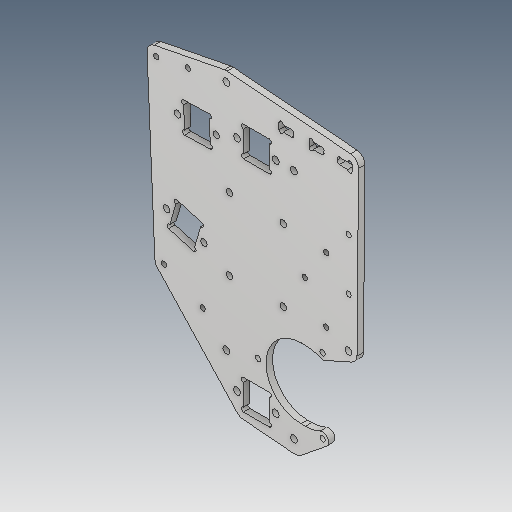
# Autodesk Inventor part: 2019スライダ側板02
Saved by Autodesk Inventor 2019.4 (Build 234330000, 330)
## iProperties
Created: 2018-05-19
Part Number: 2019スライダ側板02
Material: アルミニウム 2014-T4
Document SubType Name: Modeling
Designer: AzLIer
Density: 2.8 g/cm^3
Appearance: サテン
Mass: 80.0507 g
Surface Area: 220.985 cm^2
Volume: 28.5896 cm^3
Author: AzLIer
Autodesk Inventor part; units mm, degrees
(part 1 of 2)
ref_plane "YZ Plane" through (0, 0, 0) normal (1, 0, 0) x (0, 1, 0)
ref_plane "XZ Plane" through (0, 0, 0) normal (0, 1, 0) x (-1, 0, 0)
ref_plane "作業平面1" through (0, 0, 0) normal (0, 0, 1) x (1, 0, 0)
sketch "スケッチ1" plane through (0, 0, 0) normal (0, 0, 1) x (1, 0, 0)
  line L0 (0, 148) -> (2, 148) construction
  line L1 (2, 148) -> (2, 140) construction
  line L2 (2, 140) -> (0, 140) construction
  line L3 (0, 40) -> (0, 140) construction
  line L4 (0, 40) -> (2, 40) construction
  line L5 (2, 40) -> (2, 32) construction
  line L6 (2, 32) -> (0, 32) construction
  line L7 (0, 0) -> (0, 32) construction
  line L8 (25, 0) -> (0, 0) construction
  line L9 (25, 0) -> (25, 12) construction
  line L10 (25, 12) -> (23, 12) construction
  line L11 (23, 12) -> (23, 20) construction
  line L12 (23, 20) -> (25, 20) construction
  line L13 (25, 20) -> (25, 120) construction
  line L14 (25, 120) -> (23, 120) construction
  line L15 (23, 120) -> (23, 128) construction
  line L16 (23, 128) -> (25, 128) construction
  line L17 (25, 128) -> (25, 160) construction
  line L18 (0, 160) -> (25, 160) construction
  line L19 (0, 148) -> (0, 160) construction
  line L20 (-7.5, 150) -> (62.5, 150)
  line L21 (62.5, 150) -> (62.5, 10)
  line L22 (62.5, 10) -> (-7.5, 10)
  line L23 (-7.5, 10) -> (-7.5, 150)
  line L24 (5, -403.0972) -> (20, -403.0972) projected
  line L25 (5, -403.0972) -> (5, 396.9028) projected
  line L26 (20, 396.9028) -> (5, 396.9028) projected
  line L27 (20, -403.0972) -> (20, 396.9028) projected
  circle A0 centre (12.5, -388.0972) radius 1.5 projected
  circle A1 centre (12.5, -378.0972) radius 1.5 projected
  circle A2 centre (12.5, -398.0972) radius 1.5 projected
  circle A3 centre (12.5, 371.9028) radius 1.6 projected
  circle A4 centre (12.5, 391.9028) radius 1.6 projected
  circle A5 centre (12.5, 381.9028) radius 1.6 projected
  point P0 (2, 144)
  point P1 (23, 16)
  point P2 (-1.5, 144)
  point P3 (30, 16)
  point P4 (-1.5, 36)
  point P5 (30, 124)
  dimension "d0" = 70
  dimension "d1" = 140
  dimension "d2" = 6
  dimension "d3" = 6
  dimension "d4" = 3.5
  dimension "d5" = 6
  dimension "d7" = 20
  dimension "d8" = 20
  dimension "d167" = 10
  constraints: 8 end point, 2 horizontal alignment, 2 midpoint, 2 parallel, 2 vertical alignment, 1 horizontal, 1 perpendicular
  measures "d0" distance of L21.end L22.end
  measures "d1" distance of L20.end L21.end
  measures "d2" distance from line of L20 point (2, 144)
  measures "d3" distance from line of L22 point (23, 16)
  measures "d4" distance of point (-1.5, 144) point (2, 144)
  measures "d5" distance from line of point (-1.5, 144) L23
  measures "d7" vertical distance of point (2, 144) point (30, 124)
  measures "d8" vertical distance of point (-1.5, 36) point (30, 16)
  measures "d167" distance from line of L27 point (30, 16)
extrude "押し出し1" add sketch "スケッチ1" along normal blind 3 contours L20 L25 L22 L23 | L20 L27 L22 L25 | L20 L21 L22 L27
hole "穴1" at (-1.5, 144, 0) at (30, 16, 0) at (-1.5, 36, 0) at (30, 124, 0) direction (0, 0, 1) diameter 3.2 end through all
sketch "スケッチ2" plane through (0, 0, 3) normal (0, 0, 1) x (1, 0, 0)
  line L0 (23.3, 560) -> (23.3, -40) projected
  line L1 (-7.5, 10) -> (62.5, 10) projected
  point P0 (0, 0)
  point P1 (33.3, 40)
  dimension "d18" = 10
  dimension "d19" = 30
  measures "d18" distance from line of point (33.3, 40) L0
  measures "d19" distance from line of L1 point (33.3, 40)
hole "穴2" at (33.3, 40, 3) direction (0, 0, -1) diameter 20 end through all
sketch "スケッチ3" plane through (0, 0, 3) normal (0, 0, 1) x (1, 0, 0)
  circle A0 centre (33.3, 40) radius 10 projected
  circle A1 centre (-1.5, 36) radius 1.6 projected
  circle A2 centre (-1.5, 144) radius 1.6 projected
  circle A3 centre (30, 16) radius 1.6 projected
  circle A4 centre (30, 124) radius 1.6 projected
  line L0 (62.5, 150) -> (-7.5, 150) projected
  line L1 (-7.5, 150) -> (-7.5, 10) projected
  line L2 (-7.5, 10) -> (62.5, 10) projected
  line L3 (62.5, 10) -> (62.5, 150) projected
  line L4 (-7.5, 150) -> (-47.5, 150)
  line L5 (-47.5, 150) -> (-47.5, 10)
  line L6 (-47.5, 10) -> (-7.5, 10)
  line L7 (-7.5, 10) -> (-7.5, 150)
  point P0 (0, 0)
  dimension "d27" = 40
  constraints: 8 end point, 2 parallel, 1 horizontal, 1 perpendicular, 1 point on line
  measures "d27" distance of L6.end L5.end
extrude "押し出し2" add sketch "スケッチ3" against normal blind 3 contours L1 L6 L5 L4
sketch "スケッチ4" plane through (0, 0, 3) normal (0, 0, 1) x (1, 0, 0)
  circle A0 centre (33.3, 40) radius 10 projected
  circle A1 centre (-1.5, 36) radius 1.6 projected
  circle A2 centre (-1.5, 144) radius 1.6 projected
  circle A3 centre (30, 16) radius 1.6 projected
  circle A4 centre (30, 124) radius 1.6 projected
  line L0 (62.5, 150) -> (-47.5, 150) projected
  line L1 (-47.5, 150) -> (-47.5, 10) projected
  line L2 (-47.5, 10) -> (62.5, 10) projected
  line L3 (62.5, 10) -> (62.5, 150) projected
  line L4 (-11.5199, 142.1423) -> (-129.5092, 120.2671)
  line L5 (-131.6056, 104.3356) -> (-5.2401, 44.0714)
  circle A5 centre (-19.3858, 140.684) radius 1.6 projected
  circle A6 centre (-121.6432, 121.7254) radius 1.6 projected
  circle A7 centre (-106.8945, 124.4598) radius 1.6 projected
  circle A8 centre (-34.1345, 137.9496) radius 1.6 projected
  line L6 (-128.142, 112.8928) -> (-130.8764, 127.6414) projected
  line L7 (-128.142, 112.8928) -> (-10.1527, 134.768) projected
  line L8 (-12.8871, 149.5166) -> (-10.1527, 134.768) projected
  line L9 (-130.8764, 127.6414) -> (-12.8871, 149.5166) projected
  circle A9 centre (-12.461, 47.5151) radius 1.6 projected
  circle A10 centre (-124.3847, 100.8919) radius 1.6 projected
  circle A11 centre (-110.8456, 94.435) radius 1.6 projected
  circle A12 centre (-30.5132, 56.1243) radius 1.6 projected
  line L10 (-134.8341, 97.566) -> (-128.3772, 111.1051) projected
  line L11 (-134.8341, 97.566) -> (-8.4686, 37.3019) projected
  line L12 (-2.0117, 50.841) -> (-8.4686, 37.3019) projected
  line L13 (-128.3772, 111.1051) -> (-2.0117, 50.841) projected
  point P0 (0, 0)
  point P1 (-19.3858, 140.684)
  point P2 (-34.1345, 137.9496)
  point P3 (-30.5132, 56.1243)
  point P4 (-12.461, 47.5151)
  dimension "d147" = 15
  dimension "d148" = 20
  dimension "d150" = 8
  dimension "d151" = 8
  constraints: 4 end point, 4 midpoint, 4 point on line
  measures "d147" distance of point (-19.386, 140.684) point (-34.134, 137.95)
  measures "d148" distance of point (-12.461, 47.515) point (-30.513, 56.124)
  measures "d150" distance of point (-19.386, 140.684) L4.start
  measures "d151" distance of L5.end point (-12.461, 47.515)
hole "穴3" at (-34.1345, 137.9496, 3) at (-19.3858, 140.684, 3) at (-12.461, 47.5151, 3) at (-30.5132, 56.1243, 3) direction (0, 0, -1) diameter 2.459 end through all thread size "M3x0.5" class "6H" standard "ISO Metric profile"
sketch "スケッチ5" plane through (0, 0, 3) normal (0, 0, 1) x (1, 0, 0)
  arc A0 (43, 82) -> (43.866, 83.5) centre (43, 83) ccw projected
  line L0 (43, 82) -> (39, 82) projected
  arc A1 (37, 82) -> (39, 82) centre (38, 82) ccw projected
  line L1 (37, 82) -> (37, 85) projected
  arc A2 (39, 85) -> (37, 85) centre (38, 85) ccw projected
  line L2 (39, 85) -> (43, 85) projected
  arc A3 (43.866, 83.5) -> (43, 85) centre (43, 84) ccw projected
  arc A4 (57, 140) -> (55, 140) centre (56, 140) ccw projected
  line L3 (57, 140) -> (57, 137) projected
  arc A5 (55, 137) -> (57, 137) centre (56, 137) ccw projected
  line L4 (55, 137) -> (51, 137) projected
  arc A6 (50.134, 138.5) -> (51, 137) centre (51, 138) ccw projected
  arc A7 (51, 140) -> (50.134, 138.5) centre (51, 139) ccw projected
  line L5 (51, 140) -> (55, 140) projected
  arc A8 (25, 140) -> (23, 140) centre (24, 140) ccw projected
  line L6 (25, 140) -> (29, 140) projected
  arc A9 (29.866, 138.5) -> (29, 140) centre (29, 139) ccw projected
  arc A10 (29, 137) -> (29.866, 138.5) centre (29, 138) ccw projected
  line L7 (29, 137) -> (25, 137) projected
  arc A11 (23, 137) -> (25, 137) centre (24, 137) ccw projected
  line L8 (23, 137) -> (23, 140) projected
  arc A12 (39, 140) -> (37, 140) centre (38, 140) ccw projected
  line L9 (39, 140) -> (43, 140) projected
  arc A13 (43.866, 138.5) -> (43, 140) centre (43, 139) ccw projected
  arc A14 (43, 137) -> (43.866, 138.5) centre (43, 138) ccw projected
  line L10 (43, 137) -> (39, 137) projected
  arc A15 (37, 137) -> (39, 137) centre (38, 137) ccw projected
  line L11 (37, 137) -> (37, 140) projected
  arc A16 (57, 85) -> (55, 85) centre (56, 85) ccw projected
  line L12 (57, 85) -> (57, 82) projected
  arc A17 (55, 82) -> (57, 82) centre (56, 82) ccw projected
  line L13 (55, 82) -> (51, 82) projected
  arc A18 (50.134, 83.5) -> (51, 82) centre (51, 83) ccw projected
  arc A19 (51, 85) -> (50.134, 83.5) centre (51, 84) ccw projected
  line L14 (51, 85) -> (55, 85) projected
  arc A20 (29, 82) -> (29.866, 83.5) centre (29, 83) ccw projected
  line L15 (29, 82) -> (25, 82) projected
  arc A21 (23, 82) -> (25, 82) centre (24, 82) ccw projected
  line L16 (23, 82) -> (23, 85) projected
  arc A22 (25, 85) -> (23, 85) centre (24, 85) ccw projected
  line L17 (25, 85) -> (29, 85) projected
  arc A23 (29.866, 83.5) -> (29, 85) centre (29, 84) ccw projected
  circle A24 centre (-15, 140) radius 1.5 projected
  circle A25 centre (-15, 20) radius 1.5 projected
  line L18 (23.5, 121.4019) -> (23.5, 126.5981) projected
  arc A26 (25.4286, 126.9692) -> (23.5, 126.5981) centre (24.5, 126.5981) ccw projected
  arc A27 (25.4286, 121.0308) -> (25.4286, 126.9692) centre (25, 124) ccw projected
  arc A28 (23.5, 121.4019) -> (25.4286, 121.0308) centre (24.5, 121.4019) ccw projected
  line L19 (23.5, 13.4019) -> (23.5, 18.5981) projected
  arc A29 (25.4286, 18.9692) -> (23.5, 18.5981) centre (24.5, 18.5981) ccw projected
  arc A30 (25.4286, 13.0308) -> (25.4286, 18.9692) centre (25, 16) ccw projected
  arc A31 (23.5, 13.4019) -> (25.4286, 13.0308) centre (24.5, 13.4019) ccw projected
  circle A32 centre (-1.5, 144) radius 1.6 projected
  circle A33 centre (-1.5, 36) radius 1.6 projected
  line L20 (62.5, 150) -> (-22.5, 150) projected
  line L21 (-22.5, 150) -> (-22.5, 10) projected
  line L22 (-22.5, 10) -> (62.5, 10) projected
  line L23 (62.5, 10) -> (62.5, 150) projected
  point P0 (0, 0)
extrude "押し出し3" cut sketch "スケッチ5" against normal through all contours L3 A5 L4 A6 A7 L5 A4 | L6 A9 A10 L7 A11 L8 A8 | L9 A13 A14 L10 A15 L11 A12
sketch "スケッチ6" plane through (0, 0, 3) normal (0, 0, 1) x (1, 0, 0)
  circle A0 centre (33.3, 40) radius 10
  circle A1 centre (33.3, 40) radius 16
  circle A2 centre (55.3, 64) radius 1.6
  circle A3 centre (55.3, 16) radius 1.6
  line L0 (55.3, 64) -> (55.3, 16)
  circle A4 centre (55.3, 40) radius 1.6
  circle A5 centre (55.3, 40) radius 4.6
  point P0 (0, 0)
  dimension "d42" = 3.2
  dimension "d43" = 3.2
  dimension "d44" = 48
  dimension "d46" = 3.2
  dimension "d57" = 9.2
  dimension "d186" = 22
  constraints: 6 centre point, 2 end point, 1 coincident, 1 horizontal alignment, 1 midpoint, 1 vertical, 1 vertical alignment, 4 other
  measures "d42" diameter of A2
  measures "d43" diameter of A3
  measures "d44" distance of L0.end L0.start
  measures "d46" diameter of A4
  measures "d57" diameter of A5
  measures "d186" distance of A0.centre A4.centre
extrude "押し出し4" cut sketch "スケッチ6" against normal through all contours A2
sketch "スケッチ7" plane through (0, 0, 0) normal (0, 0, -1) x (-1, 0, 0)
  circle A0 centre (-25, 100.25) radius 1.25
  circle A1 centre (-25, 66.75) radius 1.25
  circle A2 centre (0, 100.25) radius 1.25
  circle A3 centre (0, 66.75) radius 1.5
  circle A4 centre (-25, 66.75) radius 1.5
  circle A5 centre (-25, 100.25) radius 1.5
  circle A6 centre (0, 100.25) radius 1.5
  circle A7 centre (0, 66.75) radius 1.5
  point P0 (0, 0)
  dimension "d52" = 3
  dimension "d53" = 3
  dimension "d54" = 3
  constraints: 8 centre point, 4 coincident, 1 concentric, 8 other
  measures "d52" diameter of A4
  measures "d53" diameter of A5
  measures "d54" diameter of A6
extrude "押し出し5" cut sketch "スケッチ7" against normal through all contours A0 | A1 | A2 | A3 | A4 | A5 | A6
sketch "スケッチ9" plane through (0, 0, 3) normal (0, 0, 1) x (1, 0, 0)
  circle A0 centre (55.4, 111) radius 1.25
  circle A1 centre (55.4, 87) radius 1.25
  point P0 (0, 0)
  dimension "d189" = 2.5
  dimension "d190" = 24
  constraints: 2 centre point, 1 equal radius, 1 vertical alignment, 1 other
  measures "d189" diameter of A1
  measures "d190" distance of A1.centre A0.centre
extrude "押し出し7" cut sketch "スケッチ9" against normal through all
sketch "スケッチ11" plane through (0, 0, 0) normal (0, 0, -1) x (-1, 0, 0)
  circle A0 centre (-33.3, 40) radius 10 projected
  circle A1 centre (-33.3, 53) radius 1.6
  circle A2 centre (-46.3, 40) radius 1.6
  circle A3 centre (-33.3, 27) radius 1.6
  circle A4 centre (-20.3, 40) radius 1.6
  line L0 (-46.3, 40) -> (-47.3, 40) construction
  line L1 (-46.3, 41.6) -> (-47.3, 41.6)
  line L2 (-47.3, 38.4) -> (-46.3, 38.4)
  arc A5 (-46.3, 38.4) -> (-46.3, 41.6) centre (-46.3, 40) ccw
  arc A6 (-47.3, 41.6) -> (-47.3, 38.4) centre (-47.3, 40) ccw
  line L3 (-33.3, 53) -> (-34.3, 53) construction
  line L4 (-33.3, 54.6) -> (-34.3, 54.6)
  line L5 (-34.3, 51.4) -> (-33.3, 51.4)
  arc A7 (-33.3, 51.4) -> (-33.3, 54.6) centre (-33.3, 53) ccw
  arc A8 (-34.3, 54.6) -> (-34.3, 51.4) centre (-34.3, 53) ccw
  line L6 (-20.3, 40) -> (-21.3, 40) construction
  line L7 (-20.3, 41.6) -> (-21.3, 41.6)
  line L8 (-21.3, 38.4) -> (-20.3, 38.4)
  arc A9 (-20.3, 38.4) -> (-20.3, 41.6) centre (-20.3, 40) ccw
  arc A10 (-21.3, 41.6) -> (-21.3, 38.4) centre (-21.3, 40) ccw
  line L9 (-33.3, 27) -> (-34.3, 27) construction
  line L10 (-33.3, 28.6) -> (-34.3, 28.6)
  line L11 (-34.3, 25.4) -> (-33.3, 25.4)
  arc A11 (-33.3, 25.4) -> (-33.3, 28.6) centre (-33.3, 27) ccw
  arc A12 (-34.3, 28.6) -> (-34.3, 25.4) centre (-34.3, 27) ccw
  line L12 (-33.3, 40) -> (-41.8797, 40) construction
  line L13 (-33.3, 44.2737) -> (-41.8797, 44.2737)
  line L14 (-41.8797, 35.7263) -> (-33.3, 35.7263)
  arc A13 (-33.3, 35.7263) -> (-33.3, 44.2737) centre (-33.3, 40) ccw
  arc A14 (-41.8797, 44.2737) -> (-41.8797, 35.7263) centre (-41.8797, 40) ccw
  point P0 (0, 0)
  point P1 (-46.8, 40)
  point P2 (-33.8, 53)
  point P3 (-20.8, 40)
  point P4 (-33.8, 27)
  point P5 (-37.5899, 40)
  dimension "d86" = 3.2
  dimension "d87" = 13
  dimension "d90" = 360
  dimension "d92" = 3.2
  dimension "d93" = 1
  constraints: 40 end point, 20 point on circle, 20 tangent, 14 centre point, 7 parallel, 5 midpoint, 3 equal length, 3 equal radius, 3 horizontal, 1 vertical alignment, 9 other
  measures "d86" diameter of A1
  measures "d87" distance of L3.start L12.start
  measures "d92" diameter of A6
  measures "d93" distance of L0.start L0.end
extrude "押し出し8" cut sketch "スケッチ11" against normal through all contours A14 A2 | A2 A14 | A2 L2 A6 L1 | A1 | A1 L5 A8 L4 | A3 | A3 L11 A12 L10 | A4 | A4 L8 A10 L7
sketch "スケッチ12" plane through (0, 0, 0) normal (0, 0, -1) x (-1, 0, 0)
  circle A0 centre (-33.3, 40) radius 10 projected
  line L0 (-28.9411, 31) -> (-38.6589, 31)
  line L1 (-28.9411, 49) -> (-38.6589, 49)
  arc A1 (-38.6589, 49) -> (-38.6589, 31) centre (-34.3, 40) ccw
  point P0 (0, 0)
  dimension "d96" = 18
  dimension "d98" = 1
  constraints: 4 end point, 4 point on circle, 2 horizontal, 1 centre point, 1 equal radius, 1 horizontal alignment, 1 parallel
  measures "d96" distance between parallel lines of L0 L1
  measures "d98" distance of A0.centre A1.centre
extrude "押し出し9" cut sketch "スケッチ12" against normal through all contours A0 L0 L1 | A0 L0 A1 L1
sketch "スケッチ13" plane through (0, 0, 0) normal (0, 0, -1) x (-1, 0, 0)
  line L0 (-28.9411, 31) -> (-37.6589, 31)
  arc A0 (-38.6589, 31) -> (-38.6589, 49) centre (-34.3, 40) ccw projected
  line L1 (-37.6589, 49) -> (-28.9411, 49)
  arc A1 (-37.6589, 31) -> (-28.9411, 31) centre (-33.3, 40) ccw
  arc A2 (-28.9411, 49) -> (-37.6589, 49) centre (-33.3, 40) ccw
  point P0 (0, 0)
  constraints: 4 end point, 4 point on circle, 3 centre point
extrude "押し出し10" add sketch "スケッチ13" against normal up to surface (3 mm away)
sketch "スケッチ14" plane through (0, 0, 0) normal (0, 0, -1) x (-1, 0, 0)
  arc A0 (-38.6589, 49) -> (-38.6589, 31) centre (-34.3, 40) ccw projected
  arc A1 (-28.9411, 31) -> (-28.9411, 49) centre (-33.3, 40) ccw projected
  line L0 (-33.3, 40) -> (-34.3, 40) construction
  line L1 (-33.3, 50) -> (-34.3, 50)
  line L2 (-34.3, 30) -> (-33.3, 30)
  arc A2 (-33.3, 30) -> (-33.3, 50) centre (-33.3, 40) ccw
  arc A3 (-34.3, 50) -> (-34.3, 30) centre (-34.3, 40) ccw
  line L3 (-33.3, 40) -> (-34.3, 40) construction
  line L4 (-33.3, 51.5) -> (-34.3, 51.5)
  line L5 (-34.3, 28.5) -> (-33.3, 28.5)
  arc A4 (-33.3, 28.5) -> (-33.3, 51.5) centre (-33.3, 40) ccw
  arc A5 (-34.3, 51.5) -> (-34.3, 28.5) centre (-34.3, 40) ccw
  circle A6 centre (-33.3, 40) radius 8 projected
  arc A7 (-44.2614, 39.1804) -> (-41.9476, 38.665) centre (-41.3284, 46.8961) ccw projected
  arc A8 (-41.9476, 38.665) -> (-41.8161, 37.9906) centre (-33.3, 40) ccw projected
  arc A9 (-41.8161, 37.9906) -> (-43.7672, 36.6441) centre (-38.1519, 30.5941) ccw projected
  arc A10 (-43.7672, 36.6441) -> (-43.4717, 35.8332) centre (-33.3, 40) ccw projected
  arc A11 (-43.4717, 35.8332) -> (-41.1118, 36.0581) centre (-43.0665, 44.0777) ccw projected
  arc A12 (-41.1118, 36.0581) -> (-40.7784, 35.4573) centre (-33.3, 40) ccw projected
  arc A13 (-40.7784, 35.4573) -> (-42.2179, 33.5738) centre (-35.0078, 29.5551) ccw projected
  arc A14 (-42.2179, 33.5738) -> (-41.6862, 32.8939) centre (-33.3, 40) ccw projected
  arc A15 (-41.6862, 32.8939) -> (-39.5113, 33.837) centre (-43.8486, 40.8601) ccw projected
  arc A16 (-39.5113, 33.837) -> (-39.0086, 33.3687) centre (-33.3, 40) ccw projected
  arc A17 (-39.0086, 33.3687) -> (-39.7956, 31.1326) centre (-31.6966, 29.5386) ccw projected
  arc A18 (-39.7956, 31.1326) -> (-39.0799, 30.6503) centre (-33.3, 40) ccw projected
  arc A19 (-39.0799, 30.6503) -> (-37.3028, 32.2193) centre (-43.5981, 37.5583) ccw projected
  arc A20 (-37.3028, 32.2193) -> (-36.68, 31.9292) centre (-33.3, 40) ccw projected
  arc A21 (-36.68, 31.9292) -> (-36.7375, 29.5593) centre (-28.5423, 30.5461) ccw projected
  arc A22 (-36.7375, 29.5593) -> (-35.9078, 29.3218) centre (-33.3, 40) ccw projected
  arc A23 (-35.9078, 29.3218) -> (-34.7025, 31.3631) centre (-42.3395, 34.4956) ccw projected
  arc A24 (-34.7025, 31.3631) -> (-34.0206, 31.2797) centre (-33.3, 40) ccw projected
  arc A25 (-34.0206, 31.2797) -> (-33.3429, 29.0081) centre (-25.8537, 32.479) ccw projected
  arc A26 (-33.3429, 29.0081) -> (-32.4804, 29.0386) centre (-33.3, 40) ccw projected
  arc A27 (-32.4804, 29.0386) -> (-31.965, 31.3524) centre (-40.1961, 31.9716) ccw projected
  arc A28 (-31.965, 31.3524) -> (-31.2906, 31.4839) centre (-33.3, 40) ccw projected
  arc A29 (-31.2906, 31.4839) -> (-29.9441, 29.5328) centre (-23.8941, 35.1481) ccw projected
  arc A30 (-29.9441, 29.5328) -> (-29.1332, 29.8283) centre (-33.3, 40) ccw projected
  arc A31 (-29.1332, 29.8283) -> (-29.3581, 32.1882) centre (-37.3777, 30.2335) ccw projected
  arc A32 (-29.3581, 32.1882) -> (-28.7573, 32.5216) centre (-33.3, 40) ccw projected
  arc A33 (-28.7573, 32.5216) -> (-26.8738, 31.0821) centre (-22.8551, 38.2922) ccw projected
  arc A34 (-26.8738, 31.0821) -> (-26.1939, 31.6138) centre (-33.3, 40) ccw projected
  arc A35 (-26.1939, 31.6138) -> (-27.137, 33.7887) centre (-34.1601, 29.4514) ccw projected
  arc A36 (-27.137, 33.7887) -> (-26.6687, 34.2914) centre (-33.3, 40) ccw projected
  arc A37 (-26.6687, 34.2914) -> (-24.4326, 33.5044) centre (-22.8386, 41.6034) ccw projected
  arc A38 (-24.4326, 33.5044) -> (-23.9503, 34.2201) centre (-33.3, 40) ccw projected
  arc A39 (-23.9503, 34.2201) -> (-25.5193, 35.9972) centre (-30.8583, 29.7019) ccw projected
  arc A40 (-25.5193, 35.9972) -> (-25.2292, 36.62) centre (-33.3, 40) ccw projected
  arc A41 (-25.2292, 36.62) -> (-22.8593, 36.5625) centre (-23.8461, 44.7577) ccw projected
  arc A42 (-22.8593, 36.5625) -> (-22.6218, 37.3922) centre (-33.3, 40) ccw projected
  arc A43 (-22.6218, 37.3922) -> (-24.6631, 38.5975) centre (-27.7956, 30.9605) ccw projected
  arc A44 (-24.6631, 38.5975) -> (-24.5797, 39.2794) centre (-33.3, 40) ccw projected
  arc A45 (-24.5797, 39.2794) -> (-22.3081, 39.9571) centre (-25.779, 47.4463) ccw projected
  arc A46 (-22.3081, 39.9571) -> (-22.3386, 40.8196) centre (-33.3, 40) ccw projected
  arc A47 (-22.3386, 40.8196) -> (-24.6524, 41.335) centre (-25.2716, 33.1039) ccw projected
  arc A48 (-24.6524, 41.335) -> (-24.7839, 42.0094) centre (-33.3, 40) ccw projected
  arc A49 (-24.7839, 42.0094) -> (-22.8328, 43.3559) centre (-28.4481, 49.4059) ccw projected
  arc A50 (-22.8328, 43.3559) -> (-23.1283, 44.1668) centre (-33.3, 40) ccw projected
  arc A51 (-23.1283, 44.1668) -> (-25.4882, 43.9419) centre (-23.5335, 35.9223) ccw projected
  arc A52 (-25.4882, 43.9419) -> (-25.8216, 44.5427) centre (-33.3, 40) ccw projected
  arc A53 (-25.8216, 44.5427) -> (-24.3821, 46.4262) centre (-31.5922, 50.4449) ccw projected
  arc A54 (-24.3821, 46.4262) -> (-24.9138, 47.1061) centre (-33.3, 40) ccw projected
  arc A55 (-24.9138, 47.1061) -> (-27.0887, 46.163) centre (-22.7514, 39.1399) ccw projected
  arc A56 (-27.0887, 46.163) -> (-27.5914, 46.6313) centre (-33.3, 40) ccw projected
  arc A57 (-27.5914, 46.6313) -> (-26.8044, 48.8674) centre (-34.9034, 50.4614) ccw projected
  arc A58 (-26.8044, 48.8674) -> (-27.5201, 49.3497) centre (-33.3, 40) ccw projected
  arc A59 (-27.5201, 49.3497) -> (-29.2972, 47.7807) centre (-23.0019, 42.4417) ccw projected
  arc A60 (-29.2972, 47.7807) -> (-29.92, 48.0708) centre (-33.3, 40) ccw projected
  arc A61 (-29.92, 48.0708) -> (-29.8625, 50.4407) centre (-38.0577, 49.4539) ccw projected
  arc A62 (-29.8625, 50.4407) -> (-30.6922, 50.6782) centre (-33.3, 40) ccw projected
  arc A63 (-30.6922, 50.6782) -> (-31.8975, 48.6369) centre (-24.2605, 45.5044) ccw projected
  arc A64 (-31.8975, 48.6369) -> (-32.5794, 48.7203) centre (-33.3, 40) ccw projected
  arc A65 (-32.5794, 48.7203) -> (-33.2571, 50.9919) centre (-40.7463, 47.521) ccw projected
  arc A66 (-33.2571, 50.9919) -> (-34.1196, 50.9614) centre (-33.3, 40) ccw projected
  arc A67 (-34.1196, 50.9614) -> (-34.635, 48.6476) centre (-26.4039, 48.0284) ccw projected
  arc A68 (-34.635, 48.6476) -> (-35.3094, 48.5161) centre (-33.3, 40) ccw projected
  arc A69 (-35.3094, 48.5161) -> (-36.6559, 50.4672) centre (-42.7059, 44.8519) ccw projected
  arc A70 (-36.6559, 50.4672) -> (-37.4668, 50.1717) centre (-33.3, 40) ccw projected
  arc A71 (-37.4668, 50.1717) -> (-37.2419, 47.8118) centre (-29.2223, 49.7665) ccw projected
  arc A72 (-37.2419, 47.8118) -> (-37.8427, 47.4784) centre (-33.3, 40) ccw projected
  arc A73 (-37.8427, 47.4784) -> (-39.7262, 48.9179) centre (-43.7449, 41.7078) ccw projected
  arc A74 (-39.7262, 48.9179) -> (-40.4061, 48.3862) centre (-33.3, 40) ccw projected
  arc A75 (-40.4061, 48.3862) -> (-39.463, 46.2113) centre (-32.4399, 50.5486) ccw projected
  arc A76 (-39.463, 46.2113) -> (-39.9313, 45.7086) centre (-33.3, 40) ccw projected
  arc A77 (-39.9313, 45.7086) -> (-42.1674, 46.4956) centre (-43.7614, 38.3966) ccw projected
  arc A78 (-42.1674, 46.4956) -> (-42.6497, 45.7799) centre (-33.3, 40) ccw projected
  arc A79 (-42.6497, 45.7799) -> (-41.0807, 44.0028) centre (-35.7417, 50.2981) ccw projected
  arc A80 (-41.0807, 44.0028) -> (-41.3708, 43.38) centre (-33.3, 40) ccw projected
  arc A81 (-41.3708, 43.38) -> (-43.7407, 43.4375) centre (-42.7539, 35.2423) ccw projected
  arc A82 (-43.7407, 43.4375) -> (-43.9782, 42.6078) centre (-33.3, 40) ccw projected
  arc A83 (-43.9782, 42.6078) -> (-41.9369, 41.4025) centre (-38.8044, 49.0395) ccw projected
  arc A84 (-41.9369, 41.4025) -> (-42.0203, 40.7206) centre (-33.3, 40) ccw projected
  arc A85 (-42.0203, 40.7206) -> (-44.2919, 40.0429) centre (-40.821, 32.5537) ccw projected
  arc A86 (-44.2919, 40.0429) -> (-44.2614, 39.1804) centre (-33.3, 40) ccw projected
  point P0 (0, 0)
  point P1 (-33.8, 40)
  point P2 (-33.8, 40)
  dimension "d191" = 23
  dimension "d192" = 1
  constraints: 16 end point, 8 point on circle, 8 tangent, 4 centre point, 2 horizontal, 2 midpoint, 2 parallel, 1 concentric
  measures "d191" diameter of A5
  measures "d192" distance of L0.start L3.end
extrude "押し出し12" cut sketch "スケッチ14" against normal through all contours A3 A71 A72 A73 A0 | A73 A72 A71 A3 A69 A68 A67 L1 A2 A65 A64 A63 A61 A60 A59 A1 A57 A56 A55 A53 A52 A51 A49 A48 A47 A45 A44 A43 A41 A40 A39 A37 A36 A35 A33 A32 A31 A29 A28 A27 L2 A25 A24 A23 A21 A20 A19 A0 A17 A16 A15 A13 A12 A11 A9 A8 A7 A86 A85 A84 A83 A81 A80 A79 A77 A76 A75 | A75 A76 A77 A0 | A3 A67 A68 A69 | A79 A80 A81 A0 | A83 A84 A85 A86 A7 A8 A9 A0 | A2 A63 A64 A65 | A11 A12 A13 A0 | A2 A1 A59 A60 A61 | A15 A16 A17 A0 | A1 A55 A56 A57 | A19 A20 A21 A3 | A1 A51 A52 A53 | A23 A24 A25 L2 A3 | A1 A47 A48 A49 | A1 A43 A44 A45 | A27 A28 A29 A2 | A1 A39 A40 A41 | A31 A32 A33 A1 A2 | A1 A35 A36 A37 | A6
sketch "スケッチ15" plane through (0, 0, 0) normal (0, 0, -1) x (-1, 0, 0)
  line L0 (47.5, 150) -> (-62.5, 150) projected
  line L1 (-62.5, 150) -> (-62.5, 10) projected
  line L2 (-62.5, 10) -> (47.5, 10) projected
  line L3 (47.5, 10) -> (47.5, 150) projected
  line L4 (14.8879, 112.0622) -> (15.4057, 128.0538) construction
  arc A0 (14.7909, 109.0638) -> (17.8864, 111.9651) centre (14.8879, 112.0622) ccw
  arc A1 (18.4041, 127.9567) -> (15.5028, 131.0523) centre (15.4057, 128.0538) ccw
  arc A2 (19.384, 150) -> (47.5, 25.9287) centre (155.0735, 115.5275) ccw construction
  line L5 (17.9187, 112.9646) -> (20.9172, 112.8675)
  line L6 (20.9819, 114.8665) -> (21.3055, 124.8612)
  line L7 (21.3702, 126.8602) -> (18.3718, 126.9573)
  arc A3 (20.9172, 112.8675) -> (20.9819, 114.8665) centre (20.9495, 113.867) ccw
  arc A4 (21.3055, 124.8612) -> (21.3702, 126.8602) centre (21.3378, 125.8607) ccw
  line L8 (17.8864, 111.9651) -> (17.9187, 112.9646)
  line L9 (18.3718, 126.9573) -> (18.4041, 127.9567)
  line L10 (21.1437, 119.8638) -> (15.1468, 120.058) construction
  line L11 (14.7909, 109.0638) -> (15.5028, 131.0523)
  circle A5 centre (24.1421, 119.7668) radius 1.5
  arc A6 (11.8895, 112.1593) -> (14.7909, 109.0638) centre (14.8879, 112.0622) ccw
  arc A7 (15.5028, 131.0523) -> (12.4073, 128.1509) centre (15.4057, 128.0538) ccw
  line L12 (11.9219, 113.1588) -> (8.9234, 113.2558)
  line L13 (8.9882, 115.2548) -> (9.3118, 125.2496)
  line L14 (9.3765, 127.2485) -> (12.3749, 127.1514)
  arc A8 (8.9882, 115.2548) -> (8.9234, 113.2558) centre (8.9558, 114.2553) ccw
  arc A9 (9.3765, 127.2485) -> (9.3118, 125.2496) centre (9.3441, 126.249) ccw
  line L15 (11.8895, 112.1593) -> (11.9219, 113.1588)
  line L16 (12.3749, 127.1514) -> (12.4073, 128.1509)
  line L17 (9.15, 120.2522) -> (15.1468, 120.058) construction
  circle A10 centre (6.1515, 120.3493) radius 1.5
  line L18 (24.4121, 84.9889) -> (21.5304, 84.1547)
  line L19 (26.3587, 78.265) -> (20.5953, 76.5966) construction
  line L20 (27.749, 73.4622) -> (24.9683, 83.0678)
  line L21 (14.832, 74.9281) -> (20.5953, 76.5966) construction
  arc A11 (28.3052, 71.5411) -> (27.749, 73.4622) centre (28.0271, 72.5017) ccw
  line L22 (25.4235, 70.7069) -> (28.3052, 71.5411)
  arc A12 (23.6542, 66.0304) -> (25.7016, 69.7463) centre (22.8199, 68.9121) ccw
  arc A13 (24.9683, 83.0678) -> (24.4121, 84.9889) centre (24.6902, 84.0284) ccw
  line L23 (15.7671, 82.4862) -> (15.489, 83.4468)
  arc A14 (17.5364, 87.1627) -> (15.489, 83.4468) centre (18.3707, 84.281) ccw
  arc A15 (21.2524, 85.1153) -> (17.5364, 87.1627) centre (18.3707, 84.281) ccw
  line L24 (19.6602, 69.0384) -> (16.7785, 68.2042)
  line L25 (25.7016, 69.7463) -> (25.4235, 70.7069)
  arc A16 (19.9383, 68.0779) -> (23.6542, 66.0304) centre (22.8199, 68.9121) ccw
  line L26 (22.8199, 68.9121) -> (18.3707, 84.281) construction
  line L27 (23.6542, 66.0304) -> (17.5364, 87.1627)
  line L28 (19.9383, 68.0779) -> (19.6602, 69.0384)
  circle A17 centre (29.2403, 79.0993) radius 1.5
  line L29 (21.5304, 84.1547) -> (21.2524, 85.1153)
  line L30 (12.8854, 81.652) -> (15.7671, 82.4862)
  line L31 (16.2223, 70.1253) -> (13.4416, 79.7309)
  arc A18 (12.8854, 81.652) -> (13.4416, 79.7309) centre (13.1635, 80.6914) ccw
  circle A19 centre (11.9503, 74.0939) radius 1.5
  arc A20 (16.2223, 70.1253) -> (16.7785, 68.2042) centre (16.5004, 69.1647) ccw
  line L32 (17.9187, 112.9646) -> (11.9219, 113.1588)
  line L33 (18.3718, 126.9573) -> (12.3749, 127.1514)
  line L34 (21.5304, 84.1547) -> (15.7671, 82.4862)
  line L35 (25.4235, 70.7069) -> (19.6602, 69.0384)
  arc A21 (201.0636, 258.3032) -> (63.0248, -2.9083) centre (155.0735, 115.5275) ccw projected
  line L36 (128.3772, 111.1051) -> (2.0117, 50.841) projected
  point P0 (0, 0)
  dimension "d130" = 140
  dimension "d131" = 16
  dimension "d132" = 3
  dimension "d133" = 1
  dimension "d134" = 3
  dimension "d135" = 14
  dimension "d137" = 3
  dimension "d138" = 3
  dimension "d141" = 18
  dimension "d152" = 54
  constraints: 68 end point, 35 point on circle, 22 point on line, 21 centre point, 12 symmetric about line, 5 tangent, 4 midpoint, 4 parallel, 4 perpendicular, 2 collinear, 1 concentric, 1 equal radius, 59 other
  measures "d130" radius of A2
  measures "d131" distance of L4.start L4.end
  measures "d132" radius of A0
  measures "d133" radius of A3
  measures "d134" distance of L5.start L5.end
  measures "d135" distance between parallel lines of L7 L5
  measures "d137" diameter of A5
  measures "d138" distance of L10.start A5.centre
extrude "押し出し13" cut sketch "スケッチ15" against normal through all contours A21 A10 | A10 A21 | A21 A19 | A19 A21 | L32 L12 A8 L13 A9 L14 L33 L11 | L11 L33 L7 A4 L6 A3 L5 L32 | A5 | A13 L20 A11 L22 L35 L27 L34 L18 | L27 L35 L24 A20 L31 A18 L30 L34 | A17
sketch "スケッチ18" plane through (0, 0, 3) normal (0, 0, 1) x (1, 0, 0)
  line L0 (-24.4121, 84.9889) -> (-12.8854, 81.652) projected
  arc A0 (-13.4416, 79.7309) -> (-12.8854, 81.652) centre (-13.1635, 80.6914) ccw projected
  line L1 (-13.4416, 79.7309) -> (-16.2223, 70.1253) projected
  arc A1 (-16.7785, 68.2042) -> (-16.2223, 70.1253) centre (-16.5004, 69.1647) ccw projected
  line L2 (-16.7785, 68.2042) -> (-28.3052, 71.5411) projected
  arc A2 (-27.749, 73.4622) -> (-28.3052, 71.5411) centre (-28.0271, 72.5017) ccw projected
  line L3 (-27.749, 73.4622) -> (-24.9683, 83.0678) projected
  arc A3 (-24.4121, 84.9889) -> (-24.9683, 83.0678) centre (-24.6902, 84.0284) ccw projected
  circle A4 centre (-11.9503, 74.0939) radius 1.5 projected
  circle A5 centre (-6.1515, 120.3493) radius 1.5 projected
  circle A6 centre (-24.1421, 119.7668) radius 1.5 projected
  circle A7 centre (-29.2403, 79.0993) radius 1.5 projected
  arc A8 (-9.3118, 125.2496) -> (-9.3765, 127.2485) centre (-9.3441, 126.249) ccw projected
  line L4 (-9.3118, 125.2496) -> (-8.9882, 115.2548) projected
  arc A9 (-8.9234, 113.2558) -> (-8.9882, 115.2548) centre (-8.9558, 114.2553) ccw projected
  line L5 (-8.9234, 113.2558) -> (-20.9172, 112.8675) projected
  arc A10 (-20.9819, 114.8665) -> (-20.9172, 112.8675) centre (-20.9495, 113.867) ccw projected
  line L6 (-20.9819, 114.8665) -> (-21.3055, 124.8612) projected
  arc A11 (-21.3702, 126.8602) -> (-21.3055, 124.8612) centre (-21.3378, 125.8607) ccw projected
  line L7 (-21.3702, 126.8602) -> (-9.3765, 127.2485) projected
  arc A12 (34.3, 25.4) -> (34.3, 28.6) centre (34.3, 27) ccw projected
  line L8 (34.3, 25.4) -> (33.3, 25.4) projected
  arc A13 (33.3, 28.6) -> (33.3, 25.4) centre (33.3, 27) ccw projected
  line L9 (33.3, 28.6) -> (34.3, 28.6) projected
  arc A14 (34.3, 51.4) -> (34.3, 54.6) centre (34.3, 53) ccw projected
  line L10 (34.3, 51.4) -> (33.3, 51.4) projected
  arc A15 (33.3, 54.6) -> (33.3, 51.4) centre (33.3, 53) ccw projected
  line L11 (33.3, 54.6) -> (34.3, 54.6) projected
  arc A16 (21.3, 38.4) -> (21.3, 41.6) centre (21.3, 40) ccw projected
  line L12 (21.3, 38.4) -> (20.3, 38.4) projected
  arc A17 (20.3, 41.6) -> (20.3, 38.4) centre (20.3, 40) ccw projected
  line L13 (20.3, 41.6) -> (21.3, 41.6) projected
  arc A18 (47.3, 38.4) -> (47.3, 41.6) centre (47.3, 40) ccw projected
  line L14 (47.3, 38.4) -> (46.3, 38.4) projected
  arc A19 (46.3, 41.6) -> (46.3, 38.4) centre (46.3, 40) ccw projected
  line L15 (46.3, 41.6) -> (47.3, 41.6) projected
  circle A20 centre (55.4, 111) radius 1.25 projected
  circle A21 centre (25, 100.25) radius 1.5 projected
  circle A22 centre (0, 66.75) radius 1.5 projected
  circle A23 centre (25, 66.75) radius 1.5 projected
  circle A24 centre (0, 100.25) radius 1.5 projected
  circle A25 centre (55.3, 64) radius 1.6 projected
  line L16 (23, 137) -> (23, 140) projected
  arc A26 (25, 140) -> (23, 140) centre (24, 140) ccw projected
  line L17 (25, 140) -> (29, 140) projected
  arc A27 (29.866, 138.5) -> (29, 140) centre (29, 139) ccw projected
  arc A28 (29, 137) -> (29.866, 138.5) centre (29, 138) ccw projected
  line L18 (29, 137) -> (25, 137) projected
  arc A29 (23, 137) -> (25, 137) centre (24, 137) ccw projected
  line L19 (51, 140) -> (55, 140) projected
  arc A30 (57, 140) -> (55, 140) centre (56, 140) ccw projected
  line L20 (57, 140) -> (57, 137) projected
  arc A31 (55, 137) -> (57, 137) centre (56, 137) ccw projected
  line L21 (55, 137) -> (51, 137) projected
  arc A32 (50.134, 138.5) -> (51, 137) centre (51, 138) ccw projected
  arc A33 (51, 140) -> (50.134, 138.5) centre (51, 139) ccw projected
  line L22 (37, 137) -> (37, 140) projected
  arc A34 (39, 140) -> (37, 140) centre (38, 140) ccw projected
  line L23 (39, 140) -> (43, 140) projected
  arc A35 (43.866, 138.5) -> (43, 140) centre (43, 139) ccw projected
  arc A36 (43, 137) -> (43.866, 138.5) centre (43, 138) ccw projected
  line L24 (43, 137) -> (39, 137) projected
  arc A37 (37, 137) -> (39, 137) centre (38, 137) ccw projected
  circle A38 centre (-12.461, 47.5151) radius 1.2295 projected
  circle A39 centre (-34.1345, 137.9496) radius 1.2295 projected
  circle A40 centre (-19.3858, 140.684) radius 1.2295 projected
  circle A41 centre (-30.5132, 56.1243) radius 1.2295 projected
  circle A42 centre (-1.5, 36) radius 1.6 projected
  circle A43 centre (-1.5, 144) radius 1.6 projected
  circle A44 centre (30, 16) radius 1.6 projected
  circle A45 centre (30, 124) radius 1.6 projected
  line L25 (62.5, 150) -> (-47.5, 150) projected
  line L26 (-47.5, 150) -> (-47.5, 10) projected
  line L27 (-47.5, 10) -> (62.5, 10) projected
  line L28 (62.5, 10) -> (62.5, 150) projected
  arc A46 (34.3, 30) -> (34.3, 50) centre (34.3, 40) ccw projected
  arc A47 (33.3, 50) -> (33.3, 30) centre (33.3, 40) ccw projected
  line L29 (20, -348.9108) -> (5, -348.9108) projected
  line L30 (20, -348.9108) -> (20, 451.0892) projected
  line L31 (5, 451.0892) -> (20, 451.0892) projected
  line L32 (5, -348.9108) -> (5, 451.0892) projected
  circle A48 centre (12.5, -333.9108) radius 1.5 projected
  circle A49 centre (12.5, -323.9108) radius 1.5 projected
  circle A50 centre (12.5, -343.9108) radius 1.5 projected
  circle A51 centre (12.5, 426.0892) radius 1.6 projected
  circle A52 centre (12.5, 446.0892) radius 1.6 projected
  circle A53 centre (12.5, 436.0892) radius 1.6 projected
  line L33 (6.5, 131) -> (18.5, 131)
  line L34 (18.5, 129) -> (18.5, 119)
  line L35 (18.5, 117) -> (6.5, 117)
  line L36 (6.5, 119) -> (6.5, 129)
  arc A54 (6.5, 131) -> (6.5, 129) centre (6.5, 130) ccw
  arc A55 (6.5, 119) -> (6.5, 117) centre (6.5, 118) ccw
  arc A56 (18.5, 129) -> (18.5, 131) centre (18.5, 130) ccw
  arc A57 (18.5, 117) -> (18.5, 119) centre (18.5, 118) ccw
  line L37 (30, 124) -> (30, 16)
  circle A58 centre (21.5, 124) radius 1.6
  circle A59 centre (3.5, 124) radius 1.6
  line L38 (18.5, 15) -> (6.5, 15)
  arc A60 (18.5, 15) -> (18.5, 17) centre (18.5, 16) ccw
  arc A61 (6.5, 17) -> (6.5, 15) centre (6.5, 16) ccw
  circle A62 centre (21.5, 22) radius 1.6
  line L39 (18.5, 27) -> (18.5, 17)
  circle A63 centre (3.5, 22) radius 1.6
  line L40 (6.5, 17) -> (6.5, 27)
  arc A64 (6.5, 29) -> (6.5, 27) centre (6.5, 28) ccw
  line L41 (6.5, 29) -> (18.5, 29)
  arc A65 (18.5, 27) -> (18.5, 29) centre (18.5, 28) ccw
  line L42 (34.3, 30) -> (33.3, 30) projected
  line L43 (33.3, 50) -> (34.3, 50) projected
  point P0 (0, 0)
  point P1 (18.5, 124)
  point P2 (6.5, 124)
  point P3 (18.5, 22)
  point P4 (6.5, 22)
  dimension "d168" = 14
  dimension "d169" = 12
  dimension "d170" = 2
  dimension "d171" = 11.5
  dimension "d172" = 3
  dimension "d173" = 3
  dimension "d174" = 3.2
  dimension "d177" = 102
  constraints: 18 end point, 16 point on circle, 16 point on line, 12 centre point, 4 equal radius, 3 horizontal alignment, 2 midpoint, 2 parallel, 2 vertical, 1 collinear, 1 horizontal, 1 perpendicular, 25 other
  measures "d168" distance of L33.end L35.start
  measures "d169" distance of L35.start L35.end
  measures "d170" diameter of A56
  measures "d171" distance between parallel lines of L34 L37
  measures "d172" distance from line of L36 A59.centre
  measures "d173" distance from line of L34 A58.centre
  measures "d174" diameter of A58
  measures "d177" distance of A58.centre A62.centre
extrude "押し出し15" cut sketch "スケッチ18" against normal through all contours A62 L30 | L30 A62 | A58 L30 | L30 A58 | A63 L32 | L32 A63 | A59 L32 | L32 A59 | L33 A56 L34 A57 L35 A55 L36 A54 | L38 A61 L40 A64 L41 A65 L39 A60
sketch "スケッチ20" plane through (0, 0, 0) normal (0, 0, -1) x (-1, 0, 0)
  arc A0 (-27.6372, 48.2421) -> (-28.9404, 48.9997) centre (-28.9405, 47.4997) ccw projected
  arc A1 (-27.6384, 31.7571) -> (-27.6372, 48.2421) centre (-33.3, 40) ccw projected
  arc A2 (-28.9418, 30.9997) -> (-27.6384, 31.7571) centre (-28.9417, 32.4997) ccw projected
  line L0 (-28.9418, 30.9997) -> (-37.6596, 31.0003) projected
  arc A3 (-38.9628, 31.7579) -> (-37.6596, 31.0003) centre (-37.6595, 32.5003) ccw projected
  arc A4 (-38.9616, 48.2429) -> (-38.9628, 31.7579) centre (-33.3, 40) ccw projected
  arc A5 (-37.6582, 49.0003) -> (-38.9616, 48.2429) centre (-37.6583, 47.5003) ccw projected
  line L1 (-37.6582, 49.0003) -> (-28.9404, 48.9997) projected
  circle A6 centre (-20.3, 39.999) radius 1.6 projected
  circle A7 centre (-46.3, 40.001) radius 1.6 projected
  circle A8 centre (-33.299, 53) radius 1.6 projected
  circle A9 centre (-33.301, 27) radius 1.6 projected
  line L2 (-30, 113.5) -> (-20, 113.5) projected
  line L3 (-20, 113.5) -> (-20, 53.5) projected
  line L4 (-20, 53.5) -> (-30, 53.5) projected
  line L5 (-30, 53.5) -> (-30, 80) projected
  line L6 (-30, 80) -> (-22, 80) projected
  line L7 (-22, 80) -> (-22, 87) projected
  line L8 (-22, 87) -> (-30, 87) projected
  line L9 (-30, 87) -> (-30, 113.5) projected
  circle A10 centre (-25, 100.25) radius 1.25 projected
  circle A11 centre (-25, 66.75) radius 1.25 projected
  circle A12 centre (-13.3, 39.9985) radius 1.25
  circle A13 centre (-43.2987, 57.3213) radius 1.25
  circle A14 centre (-43.3013, 22.6802) radius 1.25
  circle A15 centre (-33.301, 27) radius 3
  line L10 (-33.3, 40) -> (-35.3, 40) construction
  line L11 (-33.3, 56.3) -> (-35.3, 56.3)
  line L12 (-35.3, 23.7) -> (-33.3, 23.7)
  arc A16 (-33.3, 23.7) -> (-33.3, 56.3) centre (-33.3, 40) ccw
  arc A17 (-35.3, 56.3) -> (-35.3, 23.7) centre (-35.3, 40) ccw
  arc A18 (-41.2988, 55.7211) -> (-41.2986, 58.9211) centre (-41.2987, 57.3211) ccw projected
  line L13 (-41.2988, 55.7211) -> (-43.2988, 55.7213) projected
  arc A19 (-43.2986, 58.9213) -> (-43.2988, 55.7213) centre (-43.2987, 57.3213) ccw projected
  line L14 (-43.2986, 58.9213) -> (-41.2986, 58.9211) projected
  arc A20 (-13.2999, 41.5985) -> (-13.3001, 38.3985) centre (-13.3, 39.9985) ccw projected
  line L15 (-13.2999, 41.5985) -> (-11.2999, 41.5984) projected
  arc A21 (-11.3001, 38.3984) -> (-11.2999, 41.5984) centre (-11.3, 39.9984) ccw projected
  line L16 (-11.3001, 38.3984) -> (-13.3001, 38.3985) projected
  arc A22 (-41.3014, 21.0801) -> (-41.3012, 24.2801) centre (-41.3013, 22.6801) ccw projected
  line L17 (-41.3014, 21.0801) -> (-43.3014, 21.0802) projected
  arc A23 (-43.3012, 24.2802) -> (-43.3014, 21.0802) centre (-43.3013, 22.6802) ccw projected
  line L18 (-43.3012, 24.2802) -> (-41.3012, 24.2801) projected
  arc A24 (-41.3016, 18.0801) -> (-39.0016, 18.6962) centre (-41.3013, 22.6801) ccw projected
  line L19 (-9.0003, 36.0145) -> (-39.0016, 18.6962) projected
  arc A25 (-9.0003, 36.0145) -> (-8.9997, 43.9819) centre (-11.3, 39.9984) ccw projected
  line L20 (-38.9984, 61.3046) -> (-8.9997, 43.9819) projected
  arc A26 (-38.9984, 61.3046) -> (-41.2984, 61.9211) centre (-41.2987, 57.3211) ccw projected
  line L21 (-43.2984, 61.9213) -> (-41.2984, 61.9211) projected
  arc A27 (-43.2984, 61.9213) -> (-47.8312, 58.1066) centre (-43.2987, 57.3213) ccw projected
  line L22 (-50.8325, 40.7864) -> (-47.8312, 58.1066) projected
  arc A28 (-50.8325, 40.7864) -> (-50.8326, 39.2163) centre (-46.3, 40.001) ccw projected
  line L23 (-47.8339, 21.8955) -> (-50.8326, 39.2163) projected
  arc A29 (-47.8339, 21.8955) -> (-43.3016, 18.0802) centre (-43.3013, 22.6802) ccw projected
  line L24 (-41.3016, 18.0801) -> (-43.3016, 18.0802) projected
  point P0 (0, 0)
  point P1 (-34.3, 40)
  dimension "d194" = 2.5
  dimension "d195" = 20
  dimension "d198" = 360
  dimension "d200" = 6
  dimension "d201" = 32.6
  dimension "d202" = 2
  constraints: 8 end point, 6 centre point, 4 point on circle, 4 tangent, 1 coincident, 1 horizontal, 1 midpoint, 1 parallel, 7 other
  measures "d194" diameter of A12
  measures "d195" distance of A12.centre A1.centre
  measures "d200" diameter of A15
  measures "d201" diameter of A17
  measures "d202" distance of L10.start L10.end
extrude "押し出し16" cut sketch "スケッチ20" against normal through all contours A1 A2 L0 A3 A4 A5 L1 A0 | A6 | A7 | A8 | A9 | A16 L20 L4 | L4 L20 A16 | L20 A16 L19 L12 A17 L23 A28 L22 L11 L5 L4 | L4 L5 A16 L20 | A16 L19 | L22 A28 L23 A17 | A12 | A13 | A14 | A15
sketch "スケッチ22" plane through (0, 0, 3) normal (0, 0, 1) x (1, 0, 0)
  arc A0 (35.3, 23.7) -> (35.3, 56.3) centre (35.3, 40) ccw projected
  line L0 (35.3, 23.7) -> (33.3, 23.7) projected
  arc A1 (33.3, 56.3) -> (33.3, 23.7) centre (33.3, 40) ccw projected
  line L1 (33.3, 56.3) -> (35.3, 56.3) projected
  circle A2 centre (43.2987, 57.3213) radius 1.25 projected
  circle A3 centre (13.3, 39.9985) radius 1.25 projected
  circle A4 centre (43.3013, 22.6802) radius 1.25 projected
  circle A5 centre (3.5, 22) radius 1.6 projected
  circle A6 centre (3.5, 124) radius 1.6 projected
  arc A7 (18.5, 15) -> (18.5, 17) centre (18.5, 16) ccw projected
  line L2 (18.5, 15) -> (6.5, 15) projected
  arc A8 (6.5, 17) -> (6.5, 15) centre (6.5, 16) ccw projected
  line L3 (6.5, 17) -> (6.5, 27) projected
  arc A9 (6.5, 29) -> (6.5, 27) centre (6.5, 28) ccw projected
  line L4 (6.5, 29) -> (18.5, 29) projected
  arc A10 (18.5, 27) -> (18.5, 29) centre (18.5, 28) ccw projected
  line L5 (18.5, 27) -> (18.5, 17) projected
  arc A11 (6.5, 131) -> (6.5, 129) centre (6.5, 130) ccw projected
  line L6 (6.5, 131) -> (18.5, 131) projected
  arc A12 (18.5, 129) -> (18.5, 131) centre (18.5, 130) ccw projected
  line L7 (18.5, 129) -> (18.5, 119) projected
  arc A13 (18.5, 117) -> (18.5, 119) centre (18.5, 118) ccw projected
  line L8 (18.5, 117) -> (6.5, 117) projected
  arc A14 (6.5, 119) -> (6.5, 117) centre (6.5, 118) ccw projected
  line L9 (6.5, 119) -> (6.5, 129) projected
  circle A15 centre (21.5, 124) radius 1.6 projected
  circle A16 centre (21.5, 22) radius 1.6 projected
  line L10 (-24.4121, 84.9889) -> (-12.8854, 81.652) projected
  arc A17 (-13.4416, 79.7309) -> (-12.8854, 81.652) centre (-13.1635, 80.6914) ccw projected
  line L11 (-13.4416, 79.7309) -> (-16.2223, 70.1253) projected
  arc A18 (-16.7785, 68.2042) -> (-16.2223, 70.1253) centre (-16.5004, 69.1647) ccw projected
  line L12 (-16.7785, 68.2042) -> (-28.3052, 71.5411) projected
  arc A19 (-27.749, 73.4622) -> (-28.3052, 71.5411) centre (-28.0271, 72.5017) ccw projected
  line L13 (-27.749, 73.4622) -> (-24.9683, 83.0678) projected
  arc A20 (-24.4121, 84.9889) -> (-24.9683, 83.0678) centre (-24.6902, 84.0284) ccw projected
  circle A21 centre (-11.9503, 74.0939) radius 1.5 projected
  circle A22 centre (-6.1515, 120.3493) radius 1.5 projected
  circle A23 centre (-24.1421, 119.7668) radius 1.5 projected
  circle A24 centre (-29.2403, 79.0993) radius 1.5 projected
  arc A25 (-9.3118, 125.2496) -> (-9.3765, 127.2485) centre (-9.3441, 126.249) ccw projected
  line L14 (-9.3118, 125.2496) -> (-8.9882, 115.2548) projected
  arc A26 (-8.9234, 113.2558) -> (-8.9882, 115.2548) centre (-8.9558, 114.2553) ccw projected
  line L15 (-8.9234, 113.2558) -> (-20.9172, 112.8675) projected
  arc A27 (-20.9819, 114.8665) -> (-20.9172, 112.8675) centre (-20.9495, 113.867) ccw projected
  line L16 (-20.9819, 114.8665) -> (-21.3055, 124.8612) projected
  arc A28 (-21.3702, 126.8602) -> (-21.3055, 124.8612) centre (-21.3378, 125.8607) ccw projected
  line L17 (-21.3702, 126.8602) -> (-9.3765, 127.2485) projected
  circle A29 centre (55.4, 111) radius 1.25 projected
  circle A30 centre (55.4, 87) radius 1.25 projected
  circle A31 centre (25, 100.25) radius 1.5 projected
  circle A32 centre (0, 66.75) radius 1.5 projected
  circle A33 centre (25, 66.75) radius 1.5 projected
  circle A34 centre (0, 100.25) radius 1.5 projected
  circle A35 centre (55.3, 64) radius 1.6 projected
  line L18 (23, 137) -> (23, 140) projected
  arc A36 (25, 140) -> (23, 140) centre (24, 140) ccw projected
  line L19 (25, 140) -> (29, 140) projected
  arc A37 (29.866, 138.5) -> (29, 140) centre (29, 139) ccw projected
  arc A38 (29, 137) -> (29.866, 138.5) centre (29, 138) ccw projected
  line L20 (29, 137) -> (25, 137) projected
  arc A39 (23, 137) -> (25, 137) centre (24, 137) ccw projected
  line L21 (51, 140) -> (55, 140) projected
  arc A40 (57, 140) -> (55, 140) centre (56, 140) ccw projected
  line L22 (57, 140) -> (57, 137) projected
  arc A41 (55, 137) -> (57, 137) centre (56, 137) ccw projected
  line L23 (55, 137) -> (51, 137) projected
  arc A42 (50.134, 138.5) -> (51, 137) centre (51, 138) ccw projected
  arc A43 (51, 140) -> (50.134, 138.5) centre (51, 139) ccw projected
  line L24 (37, 137) -> (37, 140) projected
  arc A44 (39, 140) -> (37, 140) centre (38, 140) ccw projected
  line L25 (39, 140) -> (43, 140) projected
  arc A45 (43.866, 138.5) -> (43, 140) centre (43, 139) ccw projected
  arc A46 (43, 137) -> (43.866, 138.5) centre (43, 138) ccw projected
  line L26 (43, 137) -> (39, 137) projected
  arc A47 (37, 137) -> (39, 137) centre (38, 137) ccw projected
  circle A48 centre (-12.461, 47.5151) radius 1.2295 projected
  circle A49 centre (-34.1345, 137.9496) radius 1.2295 projected
  circle A50 centre (-19.3858, 140.684) radius 1.2295 projected
  circle A51 centre (-30.5132, 56.1243) radius 1.2295 projected
  circle A52 centre (-1.5, 36) radius 1.6 projected
  circle A53 centre (-1.5, 144) radius 1.6 projected
  circle A54 centre (30, 16) radius 1.6 projected
  circle A55 centre (30, 124) radius 1.6 projected
  line L27 (62.5, 150) -> (-47.5, 150) projected
  line L28 (-47.5, 150) -> (-47.5, 10) projected
  line L29 (-47.5, 10) -> (62.5, 10) projected
  line L30 (62.5, 10) -> (62.5, 150) projected
  circle A56 centre (5.0093, 83.2727) radius 5.8
  line L31 (45, 98.5) -> (45, 68.5)
  line L32 (25, 100.25) -> (25, 66.75)
  point P0 (0, 0)
  point P1 (25, 83.5)
  point P2 (45, 83.5)
  point P3 (35, 83.5)
  dimension "d220" = 20
  dimension "d221" = 10
  dimension "d229" = 30
  constraints: 4 end point, 2 coincident, 2 horizontal alignment, 2 midpoint, 2 vertical, 1 centre point, 2 other
  measures "d220" distance between parallel lines of L32 L31
  measures "d221" distance of point (45, 83.5) point (35, 83.5)
  measures "d229" distance of L31.start L31.end
hole "穴4" at (45, 98.5, 3) at (45, 68.5, 3) at (35, 83.5, 3) direction (0, 0, -1) diameter 2.459 depth 8.8 tip angle 118 thread size "M3x0.5" class "6H" standard "ISO Metric profile"